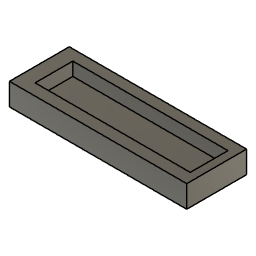
solarcad (Autodesk Fusion 360 design; units mm, degrees)
Autodesk Fusion 360 part; units mm, degrees
box "BoxPrimitive2" add length 27 width 80 height 10 placed x (0, 1, 0) y (-1, 0, 0) z (0, 0, 1) at (78.6953, 62.5055, 0)
sketch "Sketch3" plane through (0, 0, 10) normal (0, 0, 1) x (-1, 0, 0)
  line L0 (-78.6953, -89.5055) -> (1.3047, -89.5055)
  line L1 (1.3047, -89.5055) -> (1.3047, -62.5055)
  line L2 (1.3047, -62.5055) -> (-78.6953, -62.5055)
  line L3 (-78.6953, -62.5055) -> (-78.6953, -89.5055)
  line L4 (-5.0904, -84.7047) -> (-75.0904, -84.7047)
  line L5 (-75.0904, -84.7047) -> (-75.0904, -67.7047)
  line L6 (-75.0904, -67.7047) -> (-5.0904, -67.7047)
  line L7 (-5.0904, -67.7047) -> (-5.0904, -84.7047)
  dimension "d16" = 70
  dimension "d17" = 17
  constraint horizontal L4
  constraint vertical L5
  constraint horizontal L6
  constraint vertical L7
  measures "d16" distance of L4.start L4.end
  measures "d17" distance of L4.start L6.end
extrude "Extrude1" cut sketch "Sketch3" against normal blind 6 contours L4 L5 L6 L7
